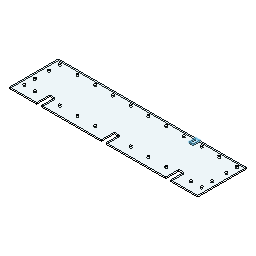
Side Panels v22 (Autodesk Fusion 360 design; units mm, degrees)
Autodesk Fusion 360 part; units mm, degrees
note: some values were not read from the file. Set by a fixed rule: which sketch regions a step uses.
sketch "Sketch1" plane through (0, 0, 0) normal (0, 0, 1) x (1, 0, 0)
  line L0 (132.5, -34.25) -> (-132.5, -34.25)
  line L1 (-132.5, -34.25) -> (-132.5, 34.25)
  line L2 (-132.5, 34.25) -> (132.5, 34.25)
  line L3 (132.5, 34.25) -> (132.5, -34.25)
  line L4 (132.5, -34.25) -> (-132.5, 34.25) construction
  line L5 (-132.5, -34.25) -> (132.5, 34.25) construction
  dimension "d1" = 68.5
  dimension "d2" = 265
  constraint horizontal L0
  constraint perpendicular L0 L1
  constraint parallel L0 L2
  constraint parallel L1 L3
  constraint coincident L4 origin
  constraint coincident L5 origin
  measures "d1" distance of L0.end L1.end
  measures "d2" distance of L1.end L2.end
extrude "Extrude1" add sketch "Sketch1" along normal blind 2
sketch "Sketch3" plane through (0, 0, 2) normal (0, 0, 1) x (-1, 0, 0)
  line L0 (-132.5, -34.25) -> (132.5, -34.25)
  line L1 (132.5, -34.25) -> (132.5, 34.25)
  line L2 (132.5, 34.25) -> (-132.5, 34.25)
  line L3 (-132.5, 34.25) -> (-132.5, -34.25)
  line L4 (94.5, 34.25) -> (87.5, 34.25)
  line L5 (87.5, 34.25) -> (87.5, 15.75)
  line L6 (87.5, 15.75) -> (94.5, 15.75)
  line L7 (94.5, 15.75) -> (94.5, 34.25)
  line L8 (3.5, 34.25) -> (-3.5, 34.25)
  line L9 (-3.5, 34.25) -> (-3.5, 15.75)
  line L10 (-3.5, 15.75) -> (3.5, 15.75)
  line L11 (3.5, 15.75) -> (3.5, 34.25)
  line L12 (-87.5, 34.25) -> (-94.5, 34.25)
  line L13 (-94.5, 34.25) -> (-94.5, 15.75)
  line L14 (-94.5, 15.75) -> (-87.5, 15.75)
  line L15 (-87.5, 15.75) -> (-87.5, 34.25)
  dimension "d9" = 18.5
  dimension "d10" = 7
  dimension "d11" = 7
  dimension "d12" = 18.5
  dimension "d13" = 38
  dimension "d14" = 84
  dimension "d15" = 7
  dimension "d16" = 18.5
  dimension "d17" = 38
  constraint horizontal L4
  constraint vertical L5
  constraint horizontal L6
  constraint vertical L7
  constraint coincident L2 L4.start
  constraint horizontal L8
  constraint vertical L9
  constraint horizontal L10
  constraint vertical L11
  constraint coincident L2 L8.start
  constraint horizontal L12
  constraint vertical L13
  constraint horizontal L14
  constraint vertical L15
  constraint coincident L2 L12.start
  measures "d9" distance of L4.start L6.end
  measures "d10" distance of L4.start L4.end
  measures "d11" distance of L8.start L8.end
  measures "d12" distance of L8.start L10.end
  measures "d13" distance of L1.end L4.start
  measures "d14" distance of L4.end L8.start
  measures "d15" distance of L12.start L12.end
  measures "d16" distance of L12.start L14.end
  measures "d17" distance of L2.end L12.end
extrude "Extrude2" cut sketch "Sketch3" against normal blind 10 contours L2 L12 L13 L14 L15 | L2 L4 L5 L6 L7 | L2 L8 L9 L10 L11
sketch "Sketch4" plane through (0, 0, 2) normal (0, 0, 1) x (-1, 0, 0)
  line L0 (87.5, 15.75) -> (87.5, 34.25)
  line L1 (87.5, 34.25) -> (3.5, 34.25)
  line L2 (3.5, 34.25) -> (3.5, 15.75)
  line L3 (3.5, 15.75) -> (-3.5, 15.75)
  line L4 (-3.5, 15.75) -> (-3.5, 34.25)
  line L5 (-3.5, 34.25) -> (-87.5, 34.25)
  line L6 (-87.5, 34.25) -> (-87.5, 15.75)
  line L7 (-87.5, 15.75) -> (-94.5, 15.75)
  line L8 (-94.5, 15.75) -> (-94.5, 34.25)
  line L9 (-94.5, 34.25) -> (-132.5, 34.25)
  line L10 (-132.5, 34.25) -> (-132.5, -34.25)
  line L11 (-132.5, -34.25) -> (132.5, -34.25)
  line L12 (132.5, -34.25) -> (132.5, 34.25)
  line L13 (132.5, 34.25) -> (94.5, 34.25)
  line L14 (94.5, 34.25) -> (94.5, 15.75)
  line L15 (94.5, 15.75) -> (87.5, 15.75)
  line L16 (-61.4253, -34.25) -> (-66.4253, -34.25)
  line L17 (-66.4253, -34.25) -> (-66.4253, -25.25)
  line L18 (-66.4253, -25.25) -> (-61.4253, -25.25)
  line L19 (-61.4253, -25.25) -> (-61.4253, -34.25)
  dimension "d20" = 5
  dimension "d21" = 9
  constraint horizontal L16
  constraint vertical L17
  constraint horizontal L18
  constraint vertical L19
  measures "d20" distance of L16.start L16.end
  measures "d21" distance of L16.start L18.end
extrude "Extrude3" cut sketch "Sketch4" against normal blind 18 contours L11 L16 L17 L18 L19
sketch "Sketch5" plane through (0, 0, 2) normal (0, 0, 1) x (-1, 0, 0)
  line L0 (-61.4253, -25.25) -> (-61.4253, -34.25)
  line L1 (-61.4253, -34.25) -> (132.5, -34.25)
  line L2 (132.5, -34.25) -> (132.5, 34.25)
  line L3 (132.5, 34.25) -> (94.5, 34.25)
  line L4 (94.5, 34.25) -> (94.5, 15.75)
  line L5 (94.5, 15.75) -> (87.5, 15.75)
  line L6 (87.5, 15.75) -> (87.5, 34.25)
  line L7 (87.5, 34.25) -> (3.5, 34.25)
  line L8 (3.5, 34.25) -> (3.5, 15.75)
  line L9 (3.5, 15.75) -> (-3.5, 15.75)
  line L10 (-3.5, 15.75) -> (-3.5, 34.25)
  line L11 (-3.5, 34.25) -> (-87.5, 34.25)
  line L12 (-87.5, 34.25) -> (-87.5, 15.75)
  line L13 (-87.5, 15.75) -> (-94.5, 15.75)
  line L14 (-94.5, 15.75) -> (-94.5, 34.25)
  line L15 (-94.5, 34.25) -> (-132.5, 34.25)
  line L16 (-132.5, 34.25) -> (-132.5, -34.25)
  line L17 (-132.5, -34.25) -> (-66.4253, -34.25)
  line L18 (-66.4253, -34.25) -> (-66.4253, -25.25)
  line L19 (-66.4253, -25.25) -> (-61.4253, -25.25)
  circle A0 centre (125.463, -29.25) radius 1.5
  circle A1 centre (-124.463, -29.25) radius 1.5
  dimension "d24" = 3
  dimension "d25" = 5
  dimension "d26" = 7.037
  dimension "d27" = 3
  dimension "d28" = 5
  dimension "d29" = 8.037
  measures "d24" diameter of A0
  measures "d25" distance of L1 A0.centre
  measures "d26" distance of L2 A0.centre
  measures "d27" diameter of A1
  measures "d28" distance of L17 A1.centre
  measures "d29" distance of L16 A1.centre
sketch "Sketch6" plane through (0, 0, 2) normal (0, 0, 1) x (1, 0, 0)
  circle A0 centre (-125.463, -20.755) radius 1.5
  line L0 (-132.5, -34.25) -> (-94.5, -34.25)
  line L1 (-132.5, 34.25) -> (-132.5, -34.25)
  circle A1 centre (124.463, -20.755) radius 1.5
  line L2 (94.5, -34.25) -> (132.5, -34.25)
  line L3 (132.5, -34.25) -> (132.5, 34.25)
  dimension "d30" = 3
  dimension "d31" = 13.495
  dimension "d32" = 7.037
  dimension "d33" = 3
  dimension "d34" = 13.495
  dimension "d35" = 8.037
  measures "d30" diameter of A0
  measures "d31" distance of A0.centre L0
  measures "d32" distance of A0.centre L1
  measures "d33" diameter of A1
  measures "d34" distance of A1.centre L2
  measures "d35" distance of A1.centre L3
extrude "Extrude4" cut sketch "Sketch5" sketch "Sketch6" against normal blind 28 contours A0 | A1 of sketch 2
sketch "Sketch7" plane through (0, 0, 0) normal (0, 0, -1) x (1, 0, 0)
  circle A0 centre (-125.463, 20.755) radius 1.5
  circle A1 centre (-125.463, -29.25) radius 1.5
  circle A2 centre (124.463, -29.25) radius 1.5
  circle A3 centre (124.463, 20.755) radius 1.5
  line L0 (61.4253, -34.25) -> (61.4253, -25.25)
  line L1 (61.4253, -25.25) -> (66.4253, -25.25)
  line L2 (66.4253, -25.25) -> (66.4253, -34.25)
  line L3 (66.4253, -34.25) -> (132.5, -34.25)
  line L4 (132.5, -34.25) -> (132.5, 34.25)
  line L5 (132.5, 34.25) -> (94.5, 34.25)
  line L6 (94.5, 34.25) -> (94.5, 15.75)
  line L7 (94.5, 15.75) -> (87.5, 15.75)
  line L8 (87.5, 15.75) -> (87.5, 34.25)
  line L9 (87.5, 34.25) -> (3.5, 34.25)
  line L10 (3.5, 34.25) -> (3.5, 15.75)
  line L11 (3.5, 15.75) -> (-3.5, 15.75)
  line L12 (-3.5, 15.75) -> (-3.5, 34.25)
  line L13 (-3.5, 34.25) -> (-87.5, 34.25)
  line L14 (-87.5, 34.25) -> (-87.5, 15.75)
  line L15 (-87.5, 15.75) -> (-94.5, 15.75)
  line L16 (-94.5, 15.75) -> (-94.5, 34.25)
  line L17 (-94.5, 34.25) -> (-132.5, 34.25)
  line L18 (-132.5, 34.25) -> (-132.5, -34.25)
  line L19 (-132.5, -34.25) -> (61.4253, -34.25)
  circle A4 centre (124.463, -14.25) radius 1.5
  circle A5 centre (124.463, 5.755) radius 1.5
  circle A6 centre (-125.463, -14.25) radius 1.5
  circle A7 centre (-125.463, 5.755) radius 1.5
  circle A8 centre (109.463, 20.755) radius 1.5
  circle A9 centre (-110.463, 20.755) radius 1.5
  circle A10 centre (99.463, -29.25) radius 1.5
  circle A11 centre (-100.463, -29.25) radius 1.5
  circle A12 centre (74.463, -29.25) radius 1.5
  circle A13 centre (-75.463, -29.25) radius 1.5
  circle A14 centre (-50.463, -29.25) radius 1.5
  circle A15 centre (-25.463, -29.25) radius 1.5
  circle A16 centre (-0.463, -29.25) radius 1.5
  circle A17 centre (24.537, -29.25) radius 1.5
  circle A18 centre (49.537, -29.25) radius 1.5
  circle A19 centre (74.463, 20.755) radius 1.5
  circle A20 centre (49.537, 20.755) radius 1.5
  circle A21 centre (24.537, 20.755) radius 1.5
  circle A22 centre (-25.463, 20.755) radius 1.5
  circle A23 centre (-50.463, 20.755) radius 1.5
  circle A24 centre (-75.463, 20.755) radius 1.5
  dimension "d38" = 3
  dimension "d39" = 15
  dimension "d40" = 3
  dimension "d41" = 15
  dimension "d42" = 3
  dimension "d43" = 3
  dimension "d44" = 15
  dimension "d45" = 15
  dimension "d46" = 3
  dimension "d47" = 15
  dimension "d48" = 3
  dimension "d49" = 15
  dimension "d50" = 3
  dimension "d51" = 25
  dimension "d52" = 3
  dimension "d53" = 25
  dimension "d54" = 3
  dimension "d55" = 25
  dimension "d56" = 3
  dimension "d57" = 25
  dimension "d60" = 3
  dimension "d61" = 3
  dimension "d62" = 3
  dimension "d64" = 25
  dimension "d65" = 25
  dimension "d66" = 25
  dimension "d72" = 3
  dimension "d78" = 3
  dimension "d79" = 25
  dimension "d81" = 25
  dimension "d82" = 3
  dimension "d83" = 3
  dimension "d84" = 3
  dimension "d85" = 3
  dimension "d86" = 3
  dimension "d87" = 3
  measures "d38" diameter of A4
  measures "d39" distance of A2.centre A4.centre
  measures "d40" diameter of A5
  measures "d41" distance of A3.centre A5.centre
  measures "d42" diameter of A6
  measures "d43" diameter of A7
  measures "d44" distance of A1.centre A6.centre
  measures "d45" distance of A0.centre A7.centre
  measures "d46" diameter of A8
  measures "d47" distance of A3.centre A8.centre
  measures "d48" diameter of A9
  measures "d49" distance of A0.centre A9.centre
  measures "d50" diameter of A10
  measures "d51" distance of A2.centre A10.centre
  measures "d52" diameter of A11
  measures "d53" distance of A1.centre A11.centre
  measures "d54" diameter of A12
  measures "d55" distance of A10.centre A12.centre
  measures "d56" diameter of A13
  measures "d57" distance of A11.centre A13.centre
  measures "d60" diameter of A14
  measures "d61" diameter of A15
  measures "d62" diameter of A16
  measures "d64" distance of A13.centre A14.centre
  measures "d65" distance of A14.centre A15.centre
  measures "d66" distance of A15.centre A16.centre
  measures "d72" diameter of A17
  measures "d78" diameter of A18
  measures "d79" distance of A17.centre A18.centre
  measures "d81" distance of A16.centre A17.centre
  measures "d82" diameter of A19
  measures "d83" diameter of A20
  measures "d84" diameter of A21
  measures "d85" diameter of A22
  measures "d86" diameter of A23
  measures "d87" diameter of A24
extrude "Extrude5" cut sketch "Sketch7" against normal blind 25 contours A4 | A5 | A6 | A7 | A8 | A9 | A10 | A11 | A12 | A13 | A14 | A15 | A16 | A17 | A18 | A19 | A20 | A21 | A22 | A23 | A24
